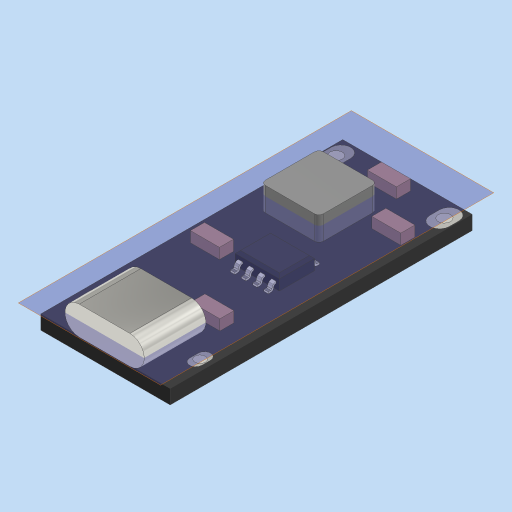
# Autodesk Inventor part: Charging_board
Saved by Autodesk Inventor 2024 (Build 280153000, 153)
## iProperties
Created: 2025-03-21
Part Number: Charging_board
Material: Generic
Document SubType Name: Modeling
Designer: XxPan
Density: 1 g/cm^3
Appearance: Default
Author: XxPan
Autodesk Inventor part; units mm, degrees
sketch "Sketch1" plane through (0, 0, 0) normal (0, 1, 0) x (-1, 0, 0)
  line L0 (7.35, 17.15) -> (-7.35, 17.15)
  line L1 (-7.35, 17.15) -> (-7.35, -17.15)
  line L2 (-7.35, -17.15) -> (7.35, -17.15)
  line L3 (7.35, -17.15) -> (7.35, 17.15)
  line L4 (10.29, 0) -> (-10.29, 0) construction
  line L5 (0, -24.01) -> (0, 24.01) construction
  point P0 (0, 0)
  dimension "d0" = 14.7
  dimension "d1" = 34.3
  constraints: 8 end point, 2 parallel, 1 horizontal, 1 perpendicular, 2 other
  measures "d0" distance of L2.end L1.end
  measures "d1" distance of L1.end L0.end
extrude "Extrusion1" add sketch "Sketch1" along normal mid plane 1.6
ref_plane "Work Plane3" through (-7.35, -0.8, 17.25) normal (0, 0, 1) x (1, 0, 0)
sketch "Sketch3" plane through (-7.35, -0.8, 17.25) normal (0, 0, 1) x (1, 0, 0)
  line L0 (2.85, 3.225) -> (11.85, 3.225) construction
  line L1 (4.475, 1.6) -> (10.225, 1.6)
  line L2 (10.225, 4.85) -> (4.475, 4.85)
  arc A0 (4.475, 4.85) -> (4.475, 1.6) centre (4.475, 3.225) ccw
  arc A1 (10.225, 1.6) -> (10.225, 4.85) centre (10.225, 3.225) ccw
  line L3 (0, 1.6) -> (14.7, 1.6) projected
  point P0 (7.35, 0.8)
  point P1 (7.35, 3.225)
  point P2 (7.35, 1.6)
  dimension "d4" = 9
  dimension "d5" = 3.25
  constraints: 8 end point, 6 point on circle, 4 tangent, 2 centre point, 2 midpoint, 2 point on line, 1 collinear, 1 horizontal, 1 parallel, 1 vertical alignment
  measures "d4" distance of L0.start L0.end
  measures "d5" diameter of A1
extrude "Extrusion2" add sketch "Sketch3" against normal blind 7
sketch "Sketch4" plane through (0, 0.8, 0) normal (0, 1, 0) x (1, 0, 0)
  line L0 (-5.05, 5.55) -> (1.55, 5.55)
  line L1 (1.55, 5.55) -> (1.55, 12.15)
  line L2 (1.55, 12.15) -> (-5.05, 12.15)
  line L3 (-5.05, 12.15) -> (-5.05, 5.55)
  line L4 (-7.35, 17.15) -> (-7.35, -17.15) projected
  line L5 (7.35, 17.15) -> (-7.35, 17.15) projected
  point P0 (0, 0)
  dimension "d8" = 6.6
  dimension "d9" = 6.6
  dimension "d10" = 2.3
  dimension "d11" = 5
  constraints: 8 end point, 2 parallel, 1 horizontal, 1 perpendicular
  measures "d8" distance of L2.end L1.end
  measures "d9" distance of L1.end L0.end
  measures "d10" distance between parallel lines of L4 L3
  measures "d11" distance between parallel lines of L5 L2
extrude "Extrusion3" add sketch "Sketch4" along normal blind 2.7
fillet "Fillet1" radius 0.5 4 edges at (1.55, 2.15, -12.15) (-5.05, 2.15, -12.15) (-5.05, 2.15, -5.55) (1.55, 2.15, -5.55)
sketch "Sketch5" plane through (0, 0.8, 0) normal (0, 1, 0) x (1, 0, 0)
  line L0 (-5.85, -1.65) -> (-2.55, -1.65)
  line L1 (-2.55, -1.65) -> (-2.55, -0.05)
  line L2 (-2.55, -0.05) -> (-5.85, -0.05)
  line L3 (-5.85, -0.05) -> (-5.85, -1.65)
  line L4 (1.2, -8.65) -> (4.5, -8.65)
  line L5 (4.5, -8.65) -> (4.5, -7.05)
  line L6 (4.5, -7.05) -> (1.2, -7.05)
  line L7 (1.2, -7.05) -> (1.2, -8.65)
  line L8 (3.05, 10.05) -> (6.35, 10.05)
  line L9 (6.35, 10.05) -> (6.35, 11.65)
  line L10 (6.35, 11.65) -> (3.05, 11.65)
  line L11 (3.05, 11.65) -> (3.05, 10.05)
  line L12 (-1.75, 14.35) -> (1.55, 14.35)
  line L13 (1.55, 14.35) -> (1.55, 15.95)
  line L14 (1.55, 15.95) -> (-1.75, 15.95)
  line L15 (-1.75, 15.95) -> (-1.75, 14.35)
  line L16 (1.55, 6.05) -> (1.55, 11.65) projected
  line L17 (2.875, -17.25) -> (2.875, -17.25) projected
  line L18 (2.875, -17.15) -> (2.875, -10.25) projected
  line L19 (2.875, -10.25) -> (2.875, -10.25) projected
  line L20 (2.875, -17.25) -> (2.875, -10.25) projected
  line L21 (2.875, -17.25) -> (2.875, -10.25) projected
  line L22 (4.5, -10.25) -> (2.875, -10.25) projected
  line L23 (-7.35, 17.15) -> (-7.35, -17.15) projected
  line L24 (7.35, -17.15) -> (7.35, 17.15) projected
  line L25 (7.35, 17.15) -> (-7.35, 17.15) projected
  line L26 (-4.55, 5.55) -> (1.05, 5.55) projected
  line L27 (2.875, -17.25) -> (2.875, -17.15) projected
  point P0 (0, 0)
  dimension "d15" = 3.3
  dimension "d16" = 1.6
  dimension "d17" = 1.6
  dimension "d18" = 1.6
  dimension "d19" = 1.6
  dimension "d20" = 3.3
  dimension "d21" = 3.3
  dimension "d22" = 3.3
  dimension "d23" = 1.5
  dimension "d24" = 1
  dimension "d25" = 1.2
  dimension "d26" = 5.5
  dimension "d27" = 1.6
  dimension "d28" = 5.6
  constraints: 32 end point, 8 parallel, 4 horizontal, 4 perpendicular, 1 collinear, 1 point on line
  measures "d15" distance of L2.end L1.end
  measures "d16" distance of L1.end L0.end
  measures "d17" distance of L6.end L4.start
  measures "d18" distance of L10.end L8.start
  measures "d19" distance of L14.end L12.start
  measures "d20" distance of L8.start L8.end
  measures "d21" distance of L5.end L6.end
  measures "d22" distance of L12.start L12.end
  measures "d23" distance between parallel lines of L23 L3
  measures "d24" distance between parallel lines of L24 L9
  measures "d25" distance between parallel lines of L25 L14
  measures "d26" distance between parallel lines of L25 L10
  measures "d27" distance between parallel lines of L22 L4
  measures "d28" distance between parallel lines of L26 L2
extrude "Extrusion4" add sketch "Sketch5" along normal blind 1.2
sketch "Sketch6" plane through (0, 0.8, 0) normal (0, 1, 0) x (1, 0, 0)
  line L0 (-1.05, -1.35) -> (3.95, -1.35)
  line L1 (3.95, -1.35) -> (3.95, 2.65)
  line L2 (3.95, 2.65) -> (-1.05, 2.65)
  line L3 (-1.05, 2.65) -> (-1.05, -1.35)
  line L4 (7.35, -17.15) -> (7.35, 17.15) projected
  line L5 (-4.55, 5.55) -> (1.05, 5.55) projected
  point P0 (0, 0)
  dimension "d31" = 5
  dimension "d32" = 4
  dimension "d33" = 3.4
  dimension "d34" = 2.9
  constraints: 8 end point, 2 parallel, 1 horizontal, 1 perpendicular
  measures "d31" distance of L2.end L1.end
  measures "d32" distance of L1.end L0.end
  measures "d33" distance between parallel lines of L4 L1
  measures "d34" distance between parallel lines of L5 L2
extrude "Extrusion5" add sketch "Sketch6" along normal blind 1.5
chamfer "Chamfer1" distance 0.3 angle 45 4 edges at (1.45, 2.3, -2.65) (3.95, 2.3, -0.65) (1.45, 2.3, 1.35) (-1.05, 2.3, -0.65)
ref_plane "Work Plane1" through (3.6, 0.8, 1.35) normal (1, 0, 0) x (0, 0, -1)
sketch "Sketch8" plane through (3.6, 0.8, 1.35) normal (1, 0, 0) x (0, 0, -1)
  line L0 (0, 0) -> (0, 1.2) projected
  line L1 (0, 0.6) -> (0, 0.3)
  line L2 (-0.3, 0) -> (-0.3, 1.2) construction
  arc A0 (0, 0.6) -> (-0.3, 0.3) centre (0, 0.3) ccw
  line L3 (0, 0.6) -> (-0.3, 0.3) construction
  line L4 (0, 0.6) -> (0.4243, 0.6) construction
  line L5 (-15.8, 0) -> (18.5, 0) projected
  arc A1 (-0.6, 0) -> (-0.3, 0.3) centre (-0.6, 0.3) ccw
  line L6 (-0.3, 0.3) -> (-0.6, 0) construction
  line L7 (-0.3, 0.3) -> (0.1243, 0.3) construction
  line L8 (-0.6, 0) -> (-0.9, 0)
  line L9 (0.2, 0.3) -> (0.2, 0.7583)
  arc A2 (0.2, 0.7583) -> (-0.5, 0.3) centre (0, 0.3) ccw
  arc A3 (-0.6, 0.2) -> (-0.5, 0.3) centre (-0.6, 0.3) ccw
  line L10 (-0.6, 0.2) -> (-0.9, 0.2)
  line L11 (-0.9, 0.2) -> (-0.9, 0)
  point P0 (1.35, -0.8)
  point P1 (0, 0.8)
  dimension "d4" = 9
  dimension "d5" = 3.25
  dimension "d41" = 0.3
  dimension "d42" = 135
  dimension "d43" = 135
  dimension "d44" = 0.3
  dimension "d45" = 0.3
  dimension "d46" = 0.3
  dimension "d47" = 0.2
  constraints: 18 end point, 8 point on circle, 4 centre point, 4 point on line, 2 equal length, 2 horizontal, 1 midpoint, 1 vertical, 3 other
  measures "d41" distance of L1.start L1.end
  measures "d42" angle of L3 L4
  measures "d43" angle of L6 L7
  measures "d44" radius of A1
  measures "d45" radius of A0
  measures "d46" distance of L6.end L8.end
  measures "d47" radial gap between concentric circles of A1 A3
extrude "Extrusion6" add sketch "Sketch8" against normal blind 0.5 contours L5 L11 L10 A3 A2 L0 A0 A1
pattern_linear "Rectangular Pattern1" count 4 spacing 1.27 along (-1, 0, 0) of "Extrusion6"
ref_plane "Work Plane2" through (-1.05, 0.8, -0.65) normal (0, 0, 1) x (1, 0, 0)
mirror "Mirror1" about plane through (-1.05, 0.8, -0.65) normal (0, 0, 1) of "Extrusion6", "Rectangular Pattern1"
sketch "Sketch9" plane through (0, 0.8, 0) normal (0, 1, 0) x (1, 0, 0)
  circle A0 centre (-6.15, -12.55) radius 0.6
  circle A1 centre (6.15, -12.55) radius 0.6
  circle A2 centre (6.15, 15.2) radius 0.7
  circle A3 centre (-6.15, 15.2) radius 0.7
  line L0 (-7.35, 17.15) -> (-7.35, -17.15) projected
  line L1 (7.35, 17.15) -> (-7.35, 17.15) projected
  line L2 (7.35, -17.15) -> (7.35, 17.15) projected
  line L3 (2.875, -17.15) -> (7.35, -17.15) projected
  point P0 (0, 0)
  dimension "d53" = 1.2
  dimension "d54" = 1.2
  dimension "d55" = 1.4
  dimension "d56" = 1.4
  dimension "d57" = 0.5
  dimension "d58" = 1.25
  dimension "d59" = 0.5
  dimension "d60" = 4
  constraints: 4 centre point, 2 horizontal alignment, 2 vertical alignment
  measures "d53" diameter of A0
  measures "d54" diameter of A1
  measures "d55" diameter of A2
  measures "d56" diameter of A3
  measures "d57" distance edge to line of A3 L0
  measures "d58" distance edge to line of A3 L1
  measures "d59" distance edge to line of A2 L2
  measures "d60" distance edge to line of A1 L3
extrude "Extrusion7" cut sketch "Sketch9" against normal through all
sketch "Sketch10" plane through (0, 0.8, 0) normal (0, 1, 0) x (1, 0, 0)
  line L0 (-6.15, -13.75) -> (-6.15, -11.35) construction
  line L1 (-5.45, -13.05) -> (-5.45, -12.05)
  line L2 (-6.85, -12.05) -> (-6.85, -13.05)
  arc A0 (-6.85, -13.05) -> (-5.45, -13.05) centre (-6.15, -13.05) ccw
  arc A1 (-5.45, -12.05) -> (-6.85, -12.05) centre (-6.15, -12.05) ccw
  circle A2 centre (-6.15, -12.55) radius 0.6 construction
  line L3 (6.15, -13.75) -> (6.15, -11.35) construction
  line L4 (6.85, -13.05) -> (6.85, -12.05)
  line L5 (5.45, -12.05) -> (5.45, -13.05)
  arc A3 (5.45, -13.05) -> (6.85, -13.05) centre (6.15, -13.05) ccw
  arc A4 (6.85, -12.05) -> (5.45, -12.05) centre (6.15, -12.05) ccw
  circle A5 centre (6.15, -12.55) radius 0.6 construction
  line L6 (-6.15, 13.55) -> (-6.15, 16.85) construction
  line L7 (-5.05, 14.65) -> (-5.05, 15.75)
  line L8 (-7.25, 15.75) -> (-7.25, 14.65)
  arc A6 (-7.25, 14.65) -> (-5.05, 14.65) centre (-6.15, 14.65) ccw
  arc A7 (-5.05, 15.75) -> (-7.25, 15.75) centre (-6.15, 15.75) ccw
  line L9 (6.15, 13.55) -> (6.15, 16.85) construction
  line L10 (7.25, 14.65) -> (7.25, 15.75)
  line L11 (5.05, 15.75) -> (5.05, 14.65)
  arc A8 (5.05, 14.65) -> (7.25, 14.65) centre (6.15, 14.65) ccw
  arc A9 (7.25, 15.75) -> (5.05, 15.75) centre (6.15, 15.75) ccw
  circle A10 centre (-6.15, 15.2) radius 0.7 construction
  circle A11 centre (6.15, 15.2) radius 0.7 construction
  point P0 (0, 0)
  dimension "d64" = 2.4
  dimension "d65" = 1.4
  dimension "d66" = 2.4
  dimension "d67" = 1.4
  dimension "d68" = 3.3
  dimension "d69" = 2.2
  dimension "d70" = 3.3
  dimension "d71" = 2.2
  constraints: 32 end point, 24 point on circle, 16 tangent, 9 centre point, 8 point on line, 5 coincident, 4 midpoint, 4 parallel, 4 vertical
  measures "d64" distance of L0.start L0.end
  measures "d65" diameter of A1
  measures "d66" distance of L3.start L3.end
  measures "d67" diameter of A4
  measures "d68" distance of L6.start L6.end
  measures "d69" diameter of A7
  measures "d70" distance of L9.start L9.end
  measures "d71" diameter of A9
surface extrude "ExtrusionSrf1" sketch "Sketch10" against normal up to surface (1.6 mm away) shown no curves A8 L10 A9 L11
surface extrude "ExtrusionSrf2" sketch "Sketch10" against normal up to surface (1.6 mm away) shown no curves A4 L5 A3 L4
surface extrude "ExtrusionSrf3" sketch "Sketch10" against normal up to surface (1.6 mm away) shown no curves A1 L2 A0 L1
surface extrude "ExtrusionSrf4" sketch "Sketch10" against normal up to surface (1.6 mm away) shown no curves A6 L7 A7 L8
split_face "Split1"
split_face "Split2"
split_face "Split3"
split_face "Split4"
ref_plane "Work Plane4" through (-2.875, 2.425, 17.25) normal (0, -1, 0) x (1, 0, 0)
equation "\"d17\" = d16"
equation "\"d18\" = d16"
equation "\"d19\" = d16"
equation "\"d20\" = d15"
equation "\"d21\" = d15"
equation "\"d22\" = d15"
body "Solid1"
body "Srf1"
body "Srf2"
body "Srf3"
body "Srf4"
